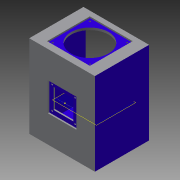
# Autodesk Inventor part: brain box bottom
Saved by Autodesk Inventor 2015 (Build 190159000, 159)
## iProperties
Created: 2014-09-09
Part Number: brain box bottom
Material: Generic
Document SubType Name: Modeling
Designer: ericd_000
Density: 1 g/cm^3
Appearance: Default
Author: ericd_000
Autodesk Inventor part; units mm, degrees
ref_plane "YZ Plane" through (0, 0, 0) normal (1, 0, 0) x (0, 1, 0)
ref_plane "XZ Plane" through (0, 0, 0) normal (0, 1, 0) x (-1, 0, 0)
ref_plane "XY Plane" through (0, 0, 0) normal (0, 0, 1) x (1, 0, 0)
sketch "Sketch1" plane through (0, 0, 0) normal (0, 1, 0) x (-1, 0, 0)
  line L0 (115, 140) -> (-115, 140)
  line L1 (-115, 140) -> (-115, -140)
  line L2 (-115, -140) -> (115, -140)
  line L3 (115, -140) -> (115, 140)
  point P0 (0, 0)
  point P1 (115, 0)
  point P2 (0, -140)
  dimension "d0" = 280
  dimension "d1" = 230
  constraints: 8 end point, 2 midpoint, 2 parallel, 1 horizontal, 1 horizontal alignment, 1 perpendicular, 1 vertical alignment
  measures "d0" distance of L2.end L0.start
  measures "d1" distance of L0.start L0.end
extrude "Extrusion1" add sketch "Sketch1" along normal blind 5
sketch "Sketch2" plane through (0, 5, 0) normal (0, 1, 0) x (1, 0, 0)
  line L0 (-115, -140) -> (115, -140)
  line L1 (115, -140) -> (115, 140)
  line L2 (115, 140) -> (-115, 140)
  line L3 (-115, 140) -> (-115, -140)
  line L4 (-107, -132) -> (107, -132)
  line L5 (107, -132) -> (107, 132)
  line L6 (107, 132) -> (-107, 132)
  line L7 (-107, 132) -> (-107, -132)
  point P0 (0, 0)
  dimension "d4" = 8
  constraints: 16 end point, 4 parallel, 2 perpendicular, 1 horizontal, 3 other
  measures "d4" distance between parallel lines of L3 L7
extrude "Extrusion2" add sketch "Sketch2" along normal blind 180
sketch "Sketch3" plane through (0, 185, 0) normal (0, 1, 0) x (1, 0, 0)
  circle A0 centre (-111, 136) radius 1.5
  circle A1 centre (111, 136) radius 1.5
  circle A2 centre (111, -136) radius 1.5
  circle A3 centre (-111, -136) radius 1.5
  line L0 (115, -140) -> (115, 140) projected
  line L1 (-115, -140) -> (115, -140) projected
  line L2 (115, 140) -> (-115, 140) projected
  line L3 (-115, 140) -> (-115, -140) projected
  point P0 (0, 0)
  dimension "d8" = 3
  dimension "d12" = 4
  dimension "d16" = 4
  dimension "d18" = 3
  dimension "d19" = 4
  dimension "d20" = 4
  dimension "d21" = 3
  dimension "d22" = 4
  dimension "d23" = 4
  dimension "d24" = 4
  dimension "d25" = 4
  dimension "d26" = 3
  constraints: 4 centre point
  measures "d8" diameter of A1
  measures "d12" distance from line of A1.centre L0
  measures "d16" distance from line of L2 A1.centre
  measures "d18" diameter of A0
  measures "d19" distance from line of L3 A0.centre
  measures "d20" distance from line of L2 A0.centre
  measures "d21" diameter of A2
  measures "d22" distance from line of L0 A2.centre
  measures "d23" distance from line of L1 A2.centre
  measures "d24" distance from line of L3 A3.centre
  measures "d25" distance from line of A3.centre L1
  measures "d26" diameter of A3
extrude "Extrusion3" cut sketch "Sketch3" against normal blind 15 contours A0 | A1 | A2 | A3
sketch "Sketch4" plane through (115, 0, 140) normal (1, 0, 0) x (0, 0, -1)
  line L0 (90, 142.5) -> (190, 142.5)
  line L1 (190, 142.5) -> (190, 42.5)
  line L2 (190, 42.5) -> (90, 42.5)
  line L3 (90, 42.5) -> (90, 142.5)
  line L4 (0, 185) -> (280, 185) projected
  line L5 (280, 0) -> (280, 185) projected
  point P0 (140, 0)
  point P1 (140, 142.5)
  point P2 (140, 185)
  point P3 (190, 92.5)
  point P4 (280, 92.5)
  dimension "d29" = 100
  dimension "d30" = 100
  constraints: 8 end point, 4 midpoint, 2 parallel, 1 horizontal, 1 horizontal alignment, 1 perpendicular, 1 vertical alignment
  measures "d29" distance of L0.start L0.end
  measures "d30" distance of L2.end L0.start
sketch "Sketch5" plane through (-115, 0, 140) normal (0, 0, 1) x (1, 0, 0)
  line L0 (230, 0) -> (230, 185) projected
  line L1 (0, 185) -> (230, 185) projected
  circle A0 centre (115, 92.5) radius 65.5
  point P0 (115, 0)
  point P1 (180.5, 92.5)
  point P2 (230, 92.5)
  point P3 (115, 158)
  point P4 (115, 185)
  dimension "d81" = 131
  constraints: 2 midpoint, 1 centre point, 1 horizontal alignment, 1 vertical alignment
  measures "d81" diameter of A0
extrude "Extrusion4" cut sketch "Sketch5" against normal blind 10
sketch "Sketch6" plane through (-115, 0, 140) normal (0, 0, 1) x (1, 0, 0)
  line L0 (49.5, 158) -> (180.5, 158)
  line L1 (180.5, 158) -> (180.5, 27)
  line L2 (180.5, 27) -> (49.5, 27)
  line L3 (49.5, 27) -> (49.5, 158)
  line L4 (40, 167.5) -> (190, 167.5)
  line L5 (190, 167.5) -> (190, 17.5)
  line L6 (190, 17.5) -> (40, 17.5)
  line L7 (40, 17.5) -> (40, 167.5)
  circle A0 centre (50, 157.5) radius 2.75
  circle A1 centre (50, 27.5) radius 2.75
  circle A2 centre (180, 157.5) radius 2.75
  circle A3 centre (180, 27.5) radius 2.75
  point P0 (115, 0)
  dimension "d35" = 9.5
  dimension "d36" = 10
  dimension "d37" = 10
  dimension "d38" = 5.5
  dimension "d41" = 130
  dimension "d44" = 130
  constraints: 16 end point, 4 centre point, 4 parallel, 2 horizontal, 2 perpendicular, 1 vertical, 9 other
  measures "d35" distance between parallel lines of L4 L0
  measures "d36" distance from line of L7 A0.centre
  measures "d37" distance from line of L4 A0.centre
  measures "d38" diameter of A0
  measures "d41" distance of A0.centre A1.centre
  measures "d44" distance of A0.centre A2.centre
extrude "Extrusion5" cut sketch "Sketch6" against normal blind 8 contours L3 A0 L0 | L0 A0 L3 | A2 L1 L0 | L0 L1 A2 | A1 L2 L3 | L3 L2 A1 | A3 L2 L1 | L1 L2 A3
sketch "Sketch7" plane through (0, 5, 0) normal (0, 1, 0) x (1, 0, 0)
  line L0 (107, 132) -> (107, -132) construction
  line L1 (107, 0) -> (-107, 0) construction
  line L2 (-107, -132) -> (-107, 132) construction
  point P0 (0, 0)
  constraints: 2 end point, 2 midpoint
ref_plane "Work Plane1" through (107, 5, 0) normal (0, 0, -1) x (-1, 0, 0)
mirror "Mirror1" about plane through (107, 5, 0) normal (0, 0, -1) of "Extrusion5"
mirror "Mirror2" about plane through (107, 5, 0) normal (0, 0, -1) of "Extrusion4"
sketch "Sketch8" plane through (0, 0, 0) normal (0, -1, 0) x (1, 0, 0)
  line L0 (35, -35) -> (-35, -35)
  line L1 (-35, -35) -> (-35, 35)
  line L2 (-35, 35) -> (35, 35)
  line L3 (35, 35) -> (35, -35)
  line L4 (50, -50) -> (-50, -50)
  line L5 (-50, -50) -> (-50, 50)
  line L6 (-50, 50) -> (50, 50)
  line L7 (50, 50) -> (50, -50)
  circle A0 centre (40, -40) radius 2.75
  circle A1 centre (40, 40) radius 2.75
  circle A2 centre (-40, -40) radius 2.75
  circle A3 centre (-40, 40) radius 2.75
  point P0 (0, 0)
  point P1 (-35, 0)
  point P2 (0, -35)
  dimension "d50" = 70
  dimension "d51" = 70
  dimension "d52" = 15
  dimension "d53" = 5.5
  dimension "d54" = 10
  dimension "d55" = 10
  dimension "d58" = 80
  dimension "d65" = 80
  constraints: 16 end point, 4 centre point, 4 parallel, 2 horizontal, 2 midpoint, 2 perpendicular, 1 horizontal alignment, 1 vertical, 1 vertical alignment, 9 other
  measures "d50" distance of L0.start L0.end
  measures "d51" distance of L0.end L1.end
  measures "d52" distance between parallel lines of L7 L3
  measures "d53" diameter of A0
  measures "d54" distance from line of L7 A0.centre
  measures "d55" distance from line of L4 A0.centre
  measures "d58" distance of A0.centre A1.centre
  measures "d65" distance of A0.centre A2.centre
extrude "Extrusion6" cut sketch "Sketch8" against normal blind 8 contours L0 L1 L2 L3 | A0 | A1 | A2 | A3
sketch "Sketch10" plane through (115, 0, -140) normal (0, 0, -1) x (-1, 0, 0)
  line L0 (190, 167.5) -> (40, 167.5)
  line L1 (40, 167.5) -> (40, 17.5)
  line L2 (40, 17.5) -> (190, 17.5)
  line L3 (190, 17.5) -> (190, 167.5)
  line L4 (0, 185) -> (230, 185) projected
  line L5 (180.5, 157.5) -> (180.5, 27.5) projected
  line L6 (177.25, 27) -> (47.25, 27) projected
  line L7 (230, 185) -> (0, 185)
  line L8 (0, 185) -> (0, 0)
  line L9 (0, 0) -> (230, 0)
  line L10 (230, 0) -> (230, 185)
  point P0 (115, 0)
  point P1 (190, 92.5)
  point P2 (180.5, 92.5)
  point P3 (180.5, 158)
  point P4 (180.5, 27)
  point P5 (115, 17.5)
  point P6 (115, 27)
  point P7 (49.5, 27)
  point P8 (177.25, 157.5)
  point P9 (177.25, 27.5)
  point P10 (177.25, 27.5)
  point P11 (47.25, 27.5)
  dimension "d72" = 150
  dimension "d73" = 150
  constraints: 16 end point, 4 parallel, 2 horizontal, 2 midpoint, 2 perpendicular, 1 horizontal alignment, 1 vertical alignment, 4 other
  measures "d72" distance of L2.end L0.start
  measures "d73" distance of L1.end L2.end
extrude "Extrusion7" add sketch "Sketch10" along normal blind 5
mirror "Mirror3" about plane through (107, 5, 0) normal (0, 0, -1) of "Extrusion7"
sketch "Sketch11" plane through (0, 0, 0) normal (0, -1, 0) x (1, 0, 0)
  line L0 (50, 50) -> (-50, 50)
  line L1 (-50, 50) -> (-50, -50)
  line L2 (-50, -50) -> (50, -50)
  line L3 (50, -50) -> (50, 50)
  line L4 (35, 35) -> (35, -35) projected
  line L5 (35, -35) -> (-35, -35) projected
  line L6 (115, 145) -> (-115, 145)
  line L7 (-115, 145) -> (-115, -145)
  line L8 (-115, -145) -> (115, -145)
  line L9 (115, -145) -> (115, 145)
  point P0 (0, 0)
  point P1 (50, 0)
  point P2 (35, 0)
  point P3 (0, -50)
  point P4 (0, -35)
  dimension "d77" = 100
  dimension "d78" = 100
  constraints: 16 end point, 4 midpoint, 4 parallel, 2 horizontal, 2 perpendicular, 1 horizontal alignment, 1 vertical alignment
  measures "d77" distance of L2.end L0.start
  measures "d78" distance of L1.end L2.end
extrude "Extrusion8" add sketch "Sketch11" along normal blind 5
body "Solid1"
